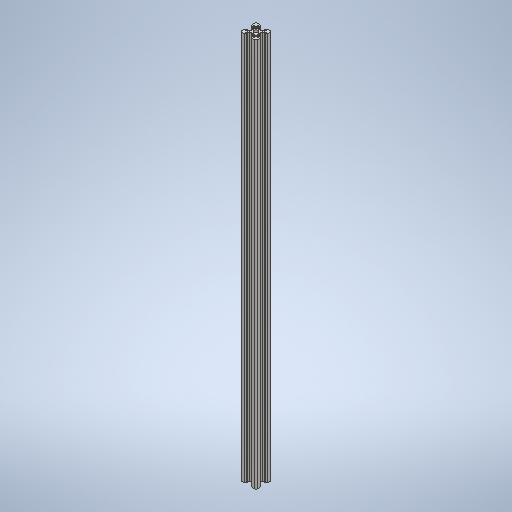
# Autodesk Inventor part: AP20x20x500
Saved by Autodesk Inventor 2025.2 (Build 292293000, 293)
## iProperties
Created: 2016-10-26
Part Number: AP20x20x500
Material: Типовые
Document SubType Name: Modeling
Designer: skhalipa
Density: 1 g/cm^3
Appearance: По умолчанию
Author: skhalipa
Autodesk Inventor part; units mm, degrees
ref_plane "YZ Plane" through (0, 0, 0) normal (1, 0, 0) x (0, 1, 0)
ref_plane "XZ Plane" through (0, 0, 0) normal (0, 1, 0) x (-1, 0, 0)
ref_plane "XY Plane" through (0, 0, 0) normal (0, 0, 1) x (1, 0, 0)
sketch "Эскиз1" plane through (0, 0, 0) normal (0, 0, 1) x (1, 0, 0)
  line L0 (-3.9516, 0.1853) -> (-3.8064, 0.0038)
  line L1 (-3.9516, -0.1778) -> (-3.8064, 0.0038)
  arc A0 (-3.9516, -0.1778) -> (-4.0064, -0.3339) centre (-3.7564, -0.3339) ccw
  line L2 (-4.0064, -0.3339) -> (-4.0064, -1.895)
  arc A1 (-4.5922, -3.3092) -> (-4.0064, -1.895) centre (-6.0064, -1.895) ccw
  line L3 (-4.5922, -3.3092) -> (-6.2863, -5.0033)
  arc A2 (-6.9934, -5.2962) -> (-6.2863, -5.0033) centre (-6.9934, -4.2962) ccw
  line L4 (-6.9934, -5.2962) -> (-7.8064, -5.2962)
  arc A3 (-8.0064, -5.0962) -> (-7.8064, -5.2962) centre (-7.8064, -5.0962) ccw
  line L5 (-8.0064, -5.0962) -> (-8.0064, -3.3262)
  arc A4 (-8.0064, -3.3262) -> (-8.4332, -3.1495) centre (-8.2564, -3.3262) ccw
  line L6 (-9.9332, -4.6495) -> (-8.4332, -3.1495)
  arc A5 (-9.9332, -4.6495) -> (-10.0064, -4.8262) centre (-9.7564, -4.8262) ccw
  line L7 (-10.0064, -4.8262) -> (-10.0064, -8.4962)
  arc A6 (-10.0064, -8.4962) -> (-8.5064, -9.9962) centre (-8.5064, -8.4962) ccw
  line L8 (-4.8364, -9.9962) -> (-8.5064, -9.9962)
  arc A7 (-4.8364, -9.9962) -> (-4.6596, -9.923) centre (-4.8364, -9.7462) ccw
  line L9 (-4.6596, -9.923) -> (-3.1596, -8.423)
  arc A8 (-3.1596, -8.423) -> (-3.3364, -7.9962) centre (-3.3364, -8.2462) ccw
  line L10 (-5.1064, -7.9962) -> (-3.3364, -7.9962)
  arc A9 (-5.3064, -7.7962) -> (-5.1064, -7.9962) centre (-5.1064, -7.7962) ccw
  line L11 (-5.3064, -6.9832) -> (-5.3064, -7.7962)
  arc A10 (-5.0135, -6.2761) -> (-5.3064, -6.9832) centre (-4.3064, -6.9832) ccw
  line L12 (-3.3194, -4.582) -> (-5.0135, -6.2761)
  arc A11 (-1.9052, -3.9962) -> (-3.3194, -4.582) centre (-1.9052, -5.9962) ccw
  line L13 (-0.3441, -3.9962) -> (-1.9052, -3.9962)
  arc A12 (-0.3441, -3.9962) -> (-0.1879, -3.9415) centre (-0.3441, -3.7462) ccw
  line L14 (-0.1879, -3.9415) -> (-0.0064, -3.7962)
  line L15 (0.1751, -3.9415) -> (-0.0064, -3.7962)
  arc A13 (0.1751, -3.9415) -> (0.3313, -3.9962) centre (0.3313, -3.7462) ccw
  line L16 (0.3313, -3.9962) -> (1.8924, -3.9962)
  arc A14 (3.3066, -4.582) -> (1.8924, -3.9962) centre (1.8924, -5.9962) ccw
  line L17 (3.3066, -4.582) -> (5.0007, -6.2761)
  arc A15 (5.2936, -6.9832) -> (5.0007, -6.2761) centre (4.2936, -6.9832) ccw
  line L18 (5.2936, -6.9832) -> (5.2936, -7.7962)
  arc A16 (5.0936, -7.9962) -> (5.2936, -7.7962) centre (5.0936, -7.7962) ccw
  line L19 (5.0936, -7.9962) -> (3.3236, -7.9962)
  arc A17 (3.3236, -7.9962) -> (3.1468, -8.423) centre (3.3236, -8.2462) ccw
  line L20 (4.6468, -9.923) -> (3.1468, -8.423)
  arc A18 (4.6468, -9.923) -> (4.8236, -9.9962) centre (4.8236, -9.7462) ccw
  line L21 (4.8236, -9.9962) -> (8.4936, -9.9962)
  arc A19 (8.4936, -9.9962) -> (9.9936, -8.4962) centre (8.4936, -8.4962) ccw
  line L22 (9.9936, -4.8262) -> (9.9936, -8.4962)
  arc A20 (9.9936, -4.8262) -> (9.9204, -4.6495) centre (9.7436, -4.8262) ccw
  line L23 (9.9204, -4.6495) -> (8.4204, -3.1495)
  arc A21 (8.4204, -3.1495) -> (7.9936, -3.3262) centre (8.2436, -3.3262) ccw
  line L24 (7.9936, -5.0962) -> (7.9936, -3.3262)
  arc A22 (7.7936, -5.2962) -> (7.9936, -5.0962) centre (7.7936, -5.0962) ccw
  line L25 (6.9806, -5.2962) -> (7.7936, -5.2962)
  arc A23 (6.2735, -5.0033) -> (6.9806, -5.2962) centre (6.9806, -4.2962) ccw
  line L26 (4.5794, -3.3092) -> (6.2735, -5.0033)
  arc A24 (3.9936, -1.895) -> (4.5794, -3.3092) centre (5.9936, -1.895) ccw
  line L27 (3.9936, -0.3339) -> (3.9936, -1.895)
  arc A25 (3.9936, -0.3339) -> (3.9388, -0.1778) centre (3.7436, -0.3339) ccw
  line L28 (3.9388, -0.1778) -> (3.7936, 0.0038)
  line L29 (3.9388, 0.1853) -> (3.7936, 0.0038)
  arc A26 (3.9388, 0.1853) -> (3.9936, 0.3415) centre (3.7436, 0.3415) ccw
  line L30 (3.9936, 0.3415) -> (3.9936, 1.9025)
  arc A27 (4.5794, 3.3168) -> (3.9936, 1.9025) centre (5.9936, 1.9025) ccw
  line L31 (4.5794, 3.3168) -> (6.2735, 5.0109)
  arc A28 (6.9806, 5.3038) -> (6.2735, 5.0109) centre (6.9806, 4.3038) ccw
  line L32 (6.9806, 5.3038) -> (7.7936, 5.3038)
  arc A29 (7.9936, 5.1038) -> (7.7936, 5.3038) centre (7.7936, 5.1038) ccw
  line L33 (7.9936, 5.1038) -> (7.9936, 3.3338)
  arc A30 (7.9936, 3.3338) -> (8.4204, 3.157) centre (8.2436, 3.3338) ccw
  line L34 (9.9204, 4.657) -> (8.4204, 3.157)
  arc A31 (9.9204, 4.657) -> (9.9936, 4.8338) centre (9.7436, 4.8338) ccw
  line L35 (9.9936, 4.8338) -> (9.9936, 8.5038)
  arc A32 (9.9936, 8.5038) -> (8.4936, 10.0038) centre (8.4936, 8.5038) ccw
  line L36 (4.8236, 10.0038) -> (8.4936, 10.0038)
  arc A33 (4.8236, 10.0038) -> (4.6468, 9.9305) centre (4.8236, 9.7538) ccw
  line L37 (4.6468, 9.9305) -> (3.1468, 8.4305)
  arc A34 (3.1468, 8.4305) -> (3.3236, 8.0038) centre (3.3236, 8.2538) ccw
  line L38 (5.0936, 8.0038) -> (3.3236, 8.0038)
  arc A35 (5.2936, 7.8038) -> (5.0936, 8.0038) centre (5.0936, 7.8038) ccw
  line L39 (5.2936, 6.9908) -> (5.2936, 7.8038)
  arc A36 (5.0007, 6.2837) -> (5.2936, 6.9908) centre (4.2936, 6.9908) ccw
  line L40 (3.3066, 4.5895) -> (5.0007, 6.2837)
  arc A37 (1.8924, 4.0038) -> (3.3066, 4.5895) centre (1.8924, 6.0038) ccw
  line L41 (0.3313, 4.0038) -> (1.8924, 4.0038)
  arc A38 (0.3313, 4.0038) -> (0.1751, 3.949) centre (0.3313, 3.7538) ccw
  line L42 (0.1751, 3.949) -> (-0.0064, 3.8038)
  line L43 (-0.1879, 3.949) -> (-0.0064, 3.8038)
  arc A39 (-0.1879, 3.949) -> (-0.3441, 4.0038) centre (-0.3441, 3.7538) ccw
  line L44 (-0.3441, 4.0038) -> (-1.9052, 4.0038)
  arc A40 (-3.3194, 4.5895) -> (-1.9052, 4.0038) centre (-1.9052, 6.0038) ccw
  line L45 (-3.3194, 4.5895) -> (-5.0135, 6.2837)
  arc A41 (-5.3064, 6.9908) -> (-5.0135, 6.2837) centre (-4.3064, 6.9908) ccw
  line L46 (-5.3064, 6.9908) -> (-5.3064, 7.8038)
  arc A42 (-5.1064, 8.0038) -> (-5.3064, 7.8038) centre (-5.1064, 7.8038) ccw
  line L47 (-5.1064, 8.0038) -> (-3.3364, 8.0038)
  arc A43 (-3.3364, 8.0038) -> (-3.1596, 8.4305) centre (-3.3364, 8.2538) ccw
  line L48 (-4.6596, 9.9305) -> (-3.1596, 8.4305)
  arc A44 (-4.6596, 9.9305) -> (-4.8364, 10.0038) centre (-4.8364, 9.7538) ccw
  line L49 (-4.8364, 10.0038) -> (-8.5064, 10.0038)
  arc A45 (-8.5064, 10.0038) -> (-10.0064, 8.5038) centre (-8.5064, 8.5038) ccw
  line L50 (-10.0064, 4.8338) -> (-10.0064, 8.5038)
  arc A46 (-10.0064, 4.8338) -> (-9.9332, 4.657) centre (-9.7564, 4.8338) ccw
  line L51 (-9.9332, 4.657) -> (-8.4332, 3.157)
  arc A47 (-8.4332, 3.157) -> (-8.0064, 3.3338) centre (-8.2564, 3.3338) ccw
  line L52 (-8.0064, 5.1038) -> (-8.0064, 3.3338)
  arc A48 (-7.8064, 5.3038) -> (-8.0064, 5.1038) centre (-7.8064, 5.1038) ccw
  line L53 (-6.9934, 5.3038) -> (-7.8064, 5.3038)
  arc A49 (-6.2863, 5.0109) -> (-6.9934, 5.3038) centre (-6.9934, 4.3038) ccw
  line L54 (-4.5922, 3.3168) -> (-6.2863, 5.0109)
  arc A50 (-4.0064, 1.9025) -> (-4.5922, 3.3168) centre (-6.0064, 1.9025) ccw
  line L55 (-4.0064, 0.3415) -> (-4.0064, 1.9025)
  arc A51 (-4.0064, 0.3415) -> (-3.9516, 0.1853) centre (-3.7564, 0.3415) ccw
  circle A52 centre (-0.0064, 0.0038) radius 2.5
  point P0 (0, 0)
  point P1 (-0.0064, 0.0038)
  dimension "d0" = 0.25
  dimension "d1" = 1.5
  dimension "d2" = 0.2
  dimension "d3" = 1
  dimension "d4" = 2
  dimension "d5" = 5
  dimension "d6" = 135
  dimension "d7" = 38.66
  dimension "d8" = 38.66
  dimension "d9" = 45
  dimension "d10" = 2
  dimension "d11" = 4.7
  dimension "d12" = 14
  dimension "d13" = 15.3
  dimension "d14" = 20
  dimension "d15" = 2.829
  dimension "d16" = 4.629
  dimension "d17" = 7.4579
  dimension "d18" = 2.829
  dimension "d19" = 4.629
  dimension "d20" = 7.4579
  dimension "d21" = 10.6
  dimension "d22" = 4.7
  dimension "d23" = 15.3
  dimension "d24" = 2.7
  dimension "d25" = 13.3
  dimension "d26" = 5.9346
  dimension "d27" = 5.9346
  dimension "d28" = 5.9346
  dimension "d29" = 5.9346
  dimension "d30" = 9.9936
  dimension "d31" = 3.7218
  dimension "d32" = 3.7271
  dimension "d33" = 5.3038
  dimension "d34" = 2.96
  dimension "d35" = 2.9647
  dimension "d36" = 2.9742
  dimension "d37" = 2.9684
  dimension "d38" = 8.0064
  dimension "d39" = 10
  dimension "d40" = 3.729
  dimension "d41" = 10
  dimension "d42" = 3.729
  constraints: 158 tangent, 112 end point, 104 point on circle, 53 centre point, 43 equal radius, 24 parallel, 3 perpendicular, 1 horizontal, 1 vertical
  measures "d0" radius of A31
  measures "d1" radius of A32
  measures "d2" radius of A29
  measures "d3" radius of A28
  measures "d4" radius of A27
  measures "d5" diameter of A52
  measures "d6" angle of L35 L34
  measures "d7" angle of L22 L29
  measures "d8" angle of L22 L28
  measures "d9" angle of L5 L34
  measures "d10" distance between parallel lines of L35 L33
  measures "d11" distance between parallel lines of L35 L39
  measures "d12" distance between parallel lines of L35 L55
  measures "d13" distance between parallel lines of L35 L46
  measures "d14" distance between parallel lines of L35 L50
  measures "d15" distance between parallel lines of L34 L31
  measures "d16" distance between parallel lines of L34 L40
  measures "d17" distance between parallel lines of L34 L37
  measures "d18" distance between parallel lines of L23 L26
  measures "d19" distance between parallel lines of L23 L17
  measures "d20" distance between parallel lines of L23 L20
  measures "d21" distance between parallel lines of L32 L25
  measures "d22" distance between parallel lines of L32 L36
  measures "d23" distance between parallel lines of L32 L21
  measures "d24" distance between parallel lines of L32 L38
  measures "d25" distance between parallel lines of L32 L19
  measures "d26" distance between parallel lines of L29 L1
  measures "d27" distance between parallel lines of L28 L0
  measures "d28" distance between parallel lines of L42 L14
  measures "d29" distance between parallel lines of L43 L15
  measures "d30" distance from line of point (0, 0) L35
  measures "d31" distance from line of point (0, 0) L34
  measures "d32" distance from line of point (0, 0) L23
  measures "d33" distance from line of point (0, 0) L32
  measures "d34" distance from line of point (0, 0) L29
  measures "d35" distance from line of point (0, 0) L28
  measures "d36" distance from line of point (0, 0) L42
  measures "d37" distance from line of point (0, 0) L15
  measures "d38" distance from line of point (0, 0) L5
  measures "d39" distance from line of A52.centre L35
  measures "d40" distance from line of A52.centre L34
  measures "d41" distance from line of point (-0.006, 0.004) L35
  measures "d42" distance from line of point (-0.006, 0.004) L34
extrude "Выдавливание1" add sketch "Эскиз1" along normal mid plane 500
